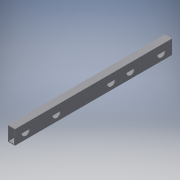
# Autodesk Inventor part: DRL Short
Saved by Autodesk Inventor 2018.2 (Build 222227000, 227)
## iProperties
Created: 2018-01-13
Part Number: DRL Short
Material: Generic
Document SubType Name: Modeling
Designer: Orangeracer
Density: 1 g/cm^3
Appearance: Default
Author: Orangeracer
Autodesk Inventor part; units mm, degrees
ref_plane "YZ Plane" through (0, 0, 0) normal (1, 0, 0) x (0, 1, 0)
ref_plane "XZ Plane" through (0, 0, 0) normal (0, 1, 0) x (-1, 0, 0)
ref_plane "XY Plane" through (0, 0, 0) normal (0, 0, 1) x (1, 0, 0)
sketch "Sketch1" plane through (0, 0, 0) normal (0, 0, 1) x (1, 0, 0)
  line L0 (0, 0) -> (25.4, 0)
  line L1 (25.4, 0) -> (25.4, -50.8)
  line L2 (25.4, -50.8) -> (0, -50.8)
  line L3 (0, -50.8) -> (0, 0)
  line L4 (22.225, -3.175) -> (3.175, -3.175)
  line L5 (3.175, -3.175) -> (3.175, -47.625)
  line L6 (3.175, -47.625) -> (22.225, -47.625)
  line L7 (22.225, -47.625) -> (22.225, -3.175)
  dimension "d0" = 25.4
  dimension "d1" = 50.8
  dimension "d2" = 3.175
  constraints: 16 end point, 4 parallel, 2 perpendicular, 1 horizontal, 3 other
  measures "d0" distance of L1.end L2.end
  measures "d1" distance of L0.end L1.end
  measures "d2" distance between parallel lines of L0 L4
extrude "Extrusion1" add sketch "Sketch1" along normal blind 559.8439
sketch "Sketch2" plane through (25.4, -50.8, 0) normal (1, 0, 0) x (0, 0, -1)
  circle A0 centre (-38.1, 25.4) radius 14.2875
  circle A1 centre (-148.1252, 25.4) radius 14.2875
  line L0 (0, 50.8) -> (0, 0) projected
  line L1 (-559.8439, 0) -> (-559.8439, 50.8) projected
  line L2 (0, 50.8) -> (-559.8439, 50.8) projected
  line L3 (0, 0) -> (-559.8439, 0) projected
  circle A2 centre (-216.7052, 25.4) radius 14.2875
  dimension "d7" = 25.4
  dimension "d8" = 25.4
  dimension "d9" = 28.575
  dimension "d10" = 28.575
  dimension "d14" = 110.0252
  dimension "d15" = 38.1
  dimension "d24" = 68.58
  dimension "d25" = 28.575
  dimension "d26" = 25.4
  constraints: 3 centre point
  measures "d7" distance from line of L2 A1.centre
  measures "d8" distance from line of L3 A0.centre
  measures "d9" diameter of A0
  measures "d10" diameter of A1
  measures "d14" distance of A0.centre A1.centre
  measures "d15" distance from line of L0 A0.centre
  measures "d24" distance of A1.centre A2.centre
  measures "d25" diameter of A2
  measures "d26" distance from line of L3 A2.centre
extrude "Extrusion2" cut sketch "Sketch2" against normal blind 254 contours A0 | A1
sketch "Sketch3" plane through (25.4, -50.8, 0) normal (1, 0, 0) x (0, 0, -1)
  circle A0 centre (-521.7439, 25.4) radius 14.2875
  circle A1 centre (-411.7188, 25.4) radius 14.2875
  line L0 (-559.8439, 0) -> (-559.8439, 50.8) projected
  line L1 (0, 50.8) -> (-559.8439, 50.8) projected
  dimension "d16" = 38.1
  dimension "d17" = 110.0252
  dimension "d18" = 25.4
  dimension "d19" = 25.4
  dimension "d20" = 28.575
  dimension "d21" = 28.575
  constraints: 2 centre point
  measures "d16" distance from line of L0 A0.centre
  measures "d17" distance of A1.centre A0.centre
  measures "d18" distance from line of L1 A1.centre
  measures "d19" distance from line of L1 A0.centre
  measures "d20" diameter of A0
  measures "d21" diameter of A1
extrude "Extrusion3" cut sketch "Sketch3" against normal blind 25.4
sketch "Sketch4" plane through (25.4, -50.8, 0) normal (1, 0, 0) x (0, 0, -1)
  circle A0 centre (-216.7052, 25.4) radius 14.2875
  circle A1 centre (-148.1252, 25.4) radius 14.2875 projected
  line L0 (0, 0) -> (-559.8439, 0) projected
  point P0 (0, 50.8)
  dimension "d27" = 68.58
  dimension "d28" = 28.575
  dimension "d29" = 25.4
  constraints: 1 centre point
  measures "d27" distance of A1.centre A0.centre
  measures "d28" diameter of A0
  measures "d29" distance from line of L0 A0.centre
extrude "Extrusion4" cut sketch "Sketch4" against normal blind 25.4 contours A0
body "Solid1"
